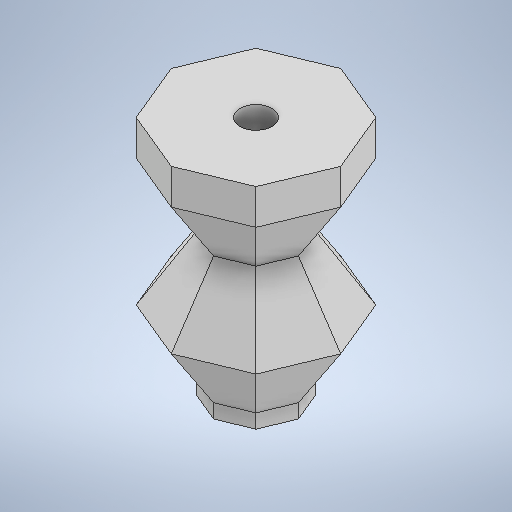
# Autodesk Inventor part: n_8
Saved by Autodesk Inventor 2025.1 (Build 291241000, 241)
## iProperties
Created: 2024-08-13
Part Number: n_8
Material: 일반
Document SubType Name: Modeling
Designer: 82103
Density: 1 g/cm^3
Appearance: 기본값
Author: 82103
Autodesk Inventor part; units mm, degrees
ref_plane "YZ Plane" through (0, 0, 0) normal (1, 0, 0) x (0, 1, 0)
ref_plane "XY Plane" through (0, 0, 0) normal (0, 0, 1) x (1, 0, 0)
sketch "스케치1" plane through (0, 0, 0) normal (0, 1, 0) x (-1, 0, 0)
  line L0 (8.4853, -8.4853) -> (0, -12)
  line L1 (0, -12) -> (-8.4853, -8.4853)
  line L2 (-8.4853, -8.4853) -> (-12, 0)
  line L3 (-12, 0) -> (-8.4853, 8.4853)
  line L4 (-8.4853, 8.4853) -> (0, 12)
  line L5 (0, 12) -> (8.4853, 8.4853)
  line L6 (8.4853, 8.4853) -> (12, 0)
  line L7 (12, 0) -> (8.4853, -8.4853)
  circle A0 centre (0, 0) radius 12 construction
  dimension "d0" = 24
  constraints: 16 end point, 2 coincident, 1 horizontal alignment, 20 other
ref_plane "작업 평면1" through (0, 9, 0) normal (0, 1, 0) x (-1, 0, 0)
sketch "스케치2" plane through (0, 9, 0) normal (0, 1, 0) x (-1, 0, 0)
  line L0 (4.2426, -4.2426) -> (0, -6)
  line L1 (0, -6) -> (-4.2426, -4.2426)
  line L2 (-4.2426, -4.2426) -> (-6, 0)
  line L3 (-6, 0) -> (-4.2426, 4.2426)
  line L4 (-4.2426, 4.2426) -> (0, 6)
  line L5 (0, 6) -> (4.2426, 4.2426)
  line L6 (4.2426, 4.2426) -> (6, 0)
  line L7 (6, 0) -> (4.2426, -4.2426)
  circle A0 centre (0, 0) radius 6 construction
  dimension "d2" = 12
  constraints: 16 end point, 2 coincident, 2 horizontal alignment, 19 other
loft "로프트1" add profiles "스케치2", "스케치1"
ref_plane "작업 평면2" through (0, 0, 0) normal (0, 1, 0) x (-1, 0, 0)
mirror "미러1" about plane through (0, 9, 0) normal (0, 1, 0) of "로프트1"
mirror "미러2" about plane through (0, 0, 0) normal (0, 1, 0) of "로프트1"
shell "쉘1" thickness 0.5 removed faces 0 ; own thickness 2 on faces at (-3.8891, -1.5, -9.3891) (-9.3891, -1.5, -3.8891) (-9.3891, -1.5, 3.8891) (-3.8891, -1.5, 9.3891) (3.8891, -1.5, 9.3891) (9.3891, -1.5, 3.8891) (9.3891, -1.5, -3.8891) (3.8891, -1.5, -9.3891) (3.8891, 16.5, -9.3891) (-3.8891, 16.5, -9.3891) (-9.3891, 16.5, -3.8891) (9.3891, 16.5, -3.8891) (-9.3891, 16.5, 3.8891) (-3.8891, 16.5, 9.3891) (3.8891, 16.5, 9.3891) (9.3891, 16.5, 3.8891)
sketch "스케치3" plane through (-4.2426, -9, -4.2426) normal (0, -1, 0) x (0.9238795, 0, -0.3826834)
  line L0 (0, 0) -> (4.5922, 0) projected
  line L1 (4.5922, 0) -> (7.8394, 3.2472) projected
  line L2 (7.8394, 3.2472) -> (7.8394, 7.8394) projected
  line L3 (7.8394, 7.8394) -> (4.5922, 11.0866) projected
  line L4 (4.5922, 11.0866) -> (0, 11.0866) projected
  line L5 (0, 11.0866) -> (-3.2472, 7.8394) projected
  line L6 (-3.2472, 7.8394) -> (-3.2472, 3.2472) projected
  line L7 (-3.2472, 3.2472) -> (0, 0) projected
  point P0 (2.2961, 5.5433)
extrude "돌출1" add sketch "스케치3" along normal blind 2
sketch "스케치4" plane through (-8.4853, 18, -8.4853) normal (0, 1, 0) x (0.9238795, 0, -0.3826834)
  line L0 (0, 0) -> (9.1844, 0) projected
  line L1 (-6.4944, -6.4944) -> (0, 0) projected
  line L2 (-6.4944, -15.6788) -> (-6.4944, -6.4944) projected
  line L3 (0, -22.1731) -> (-6.4944, -15.6788) projected
  line L4 (9.1844, -22.1731) -> (0, -22.1731) projected
  line L5 (15.6788, -15.6788) -> (9.1844, -22.1731) projected
  line L6 (15.6788, -6.4944) -> (15.6788, -15.6788) projected
  line L7 (9.1844, 0) -> (15.6788, -6.4944) projected
  point P0 (4.5922, -11.0866)
extrude "돌출2" add sketch "스케치4" along normal blind 5
sketch "스케치5" plane through (-8.4853, 23, -8.4853) normal (0, 1, 0) x (0.9238795, 0, -0.3826834)
  circle A0 centre (4.5922, -11.0866) radius 2.25
  dimension "d14" = 4.5
  constraints: 1 centre point, 1 coincident
  measures "d14" diameter of A0
extrude "돌출3" cut sketch "스케치5" against normal blind 6
